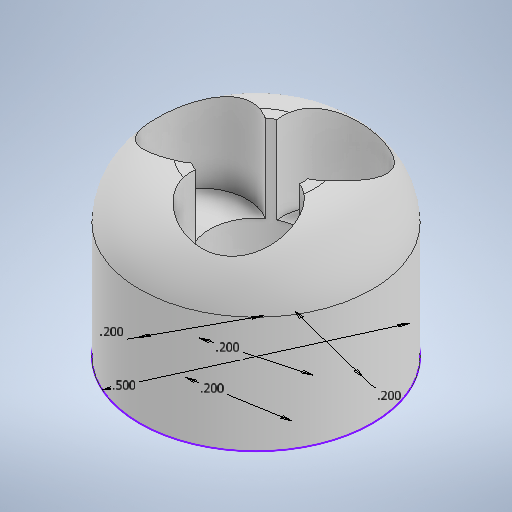
# Autodesk Inventor part: PluckTool
Saved by Autodesk Inventor 2025.1 (Build 291241000, 241)
## iProperties
Created: 2025-12-15
Part Number: PluckTool
Material: Generic
Document SubType Name: Modeling
Designer: Juxin
Density: 1 g/cm^3
Appearance: Default
Author: Juxin
Autodesk Inventor part; units mm, degrees
ref_plane "YZ Plane" through (0, 0, 0) normal (1, 0, 0) x (0, 1, 0)
ref_plane "XZ Plane" through (0, 0, 0) normal (0, 1, 0) x (-1, 0, 0)
ref_plane "XY Plane" through (0, 0, 0) normal (0, 0, 1) x (1, 0, 0)
sketch "Sketch1" plane through (0, 0, 0) normal (0, 1, 0) x (-1, 0, 0)
  circle A0 centre (0, -17.2028) radius 2.54
  circle A1 centre (0.1552, -22.2805) radius 2.54
  line L0 (0, -17.2028) -> (4.826, -17.2028) construction
  circle A2 centre (4.475, -19.6072) radius 2.54
  circle A3 centre (1.5434, -19.6969) radius 2.54
  circle A4 centre (1.5434, -19.6969) radius 6.35
  line L1 (0.1552, -22.2805) -> (0, -17.2028)
  line L2 (4.475, -19.6072) -> (0, -17.2028)
  line L3 (4.475, -19.6072) -> (0.1552, -22.2805)
  line L4 (2.3151, -20.9439) -> (0, -17.2028)
  line L5 (0.1552, -22.2805) -> (2.2375, -18.405)
  line L6 (0.0776, -19.7417) -> (4.475, -19.6072)
  point P0 (3.0726, -21.725)
  point P1 (2.6762, -21.9703)
  point P2 (-0.9776, -20.0071)
  point P3 (-0.9918, -19.5412)
  point P4 (2.5352, -17.3585)
  point P5 (2.9458, -17.5791)
  dimension "d3" = 5.08
  dimension "d7" = 5.08
  dimension "d8" = 12.7
  dimension "d14" = 5.08
  dimension "d15" = 5.08
  constraints: 14 end point, 5 centre point, 3 equal radius, 3 midpoint, 1 horizontal
  measures "d3" diameter of A0
  measures "d7" diameter of A3
  measures "d8" diameter of A4
  measures "d14" diameter of A2
  measures "d15" diameter of A1
extrude "Extrusion1" add sketch "Sketch1" along normal blind 4.7625 contours A0 A3 L2 L1 | L1 L4 A3 | A3 L1 L3 A1 | A2 A3 L3 L2 | A3 L4 L2 | A3 L5 L1 | L2 L6 A3 | A3 L3 L5 | L6 L3 A3 | A4
extrude "Extrusion2" add sketch "Sketch1" along normal blind 9.525
fillet "Fillet1" radius 3.175 1 edges at (4.8066, 9.525, -19.6969)
body "Solid1"
